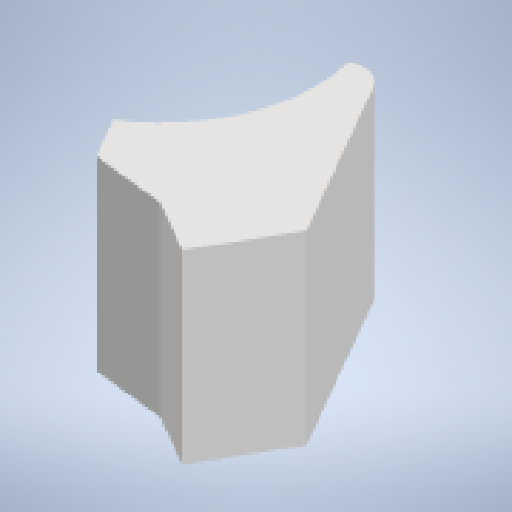
# Autodesk Inventor part: base_backwall_setter_under
Saved by Autodesk Inventor 2024.1 (Build 281209000, 209)
## iProperties
Created: 2025-01-18
Part Number: base_backwall_setter_under
Material: 一般
Document SubType Name: Modeling
Designer: hibik
Density: 1 g/cm^3
Appearance: 既定
Author: hibik
Autodesk Inventor part; units mm, degrees
ref_plane "YZ Plane" through (0, 0, 0) normal (1, 0, 0) x (0, 1, 0)
ref_plane "XZ Plane" through (0, 0, 0) normal (0, 1, 0) x (-1, 0, 0)
ref_plane "XY Plane" through (0, 0, 0) normal (0, 0, 1) x (1, 0, 0)
sketch "スケッチ2" plane through (0, 0, 0) normal (0, 1, 0) x (-1, 0, 0)
  line L0 (0, 0) -> (-8.6603, -15)
  line L1 (-8.6603, -15) -> (11.3397, -49.641)
  line L2 (73.7428, 0) -> (-22.3941, 0) projected
  line L3 (11.3397, -49.641) -> (5.9252, -52.7671) construction
  line L4 (0, 0) -> (-6.6711, 3.8516) construction
  line L5 (11.3397, -49.641) -> (24.3301, -42.141)
  line L6 (24.3301, -42.141) -> (0, 0)
  line L7 (0, 0) -> (8.2272, -4.75)
  line L8 (8.2272, -4.75) -> (-3.1754, -24.5)
  line L9 (-2.5935, -25.5079) -> (9.1002, -5.254)
  line L10 (9.1002, -5.254) -> (8.2272, -4.75)
  line L11 (-3.1754, -24.5) -> (2.5403, -27.8)
  line L12 (2.5403, -27.8) -> (12.2903, -10.9125)
  line L13 (12.2903, -10.9125) -> (6.5746, -7.6125)
  line L14 (6.5746, -7.6125) -> (-3.1754, -24.5)
  line L15 (11.3397, -49.641) -> (31.9282, -37.7543)
  line L16 (31.9282, -37.7543) -> (38.6416, -26.1264)
  line L17 (6.3397, -40.9808) -> (21.9282, -31.9808) construction
  line L18 (21.9282, -31.9808) -> (31.9282, -37.7543)
  line L19 (12.2903, -10.9125) -> (38.6416, -26.1264)
  line L20 (38.6416, -26.1264) -> (3.5066, -26.1264)
  line L21 (0, 0) -> (21.3397, 36.9615)
  line L22 (21.3397, 36.9615) -> (15.2136, 40.4985)
  line L23 (-0.5996, -1.0385) -> (60.009, -1.0385)
  circle A0 centre (21.3397, -13.5385) radius 12.5 construction
  circle A1 centre (21.3397, -13.5385) radius 10.5 construction
  circle A2 centre (20.5151, -34.5223) radius 10.5 construction
  circle A3 centre (20.5151, -34.5223) radius 11.5 construction
  circle A4 centre (20.5151, -34.5223) radius 12.5
  line L24 (8.3719, -37.4876) -> (11.3397, -49.641)
  line L25 (-2.3094, -23) -> (12.6388, -48.891)
  point P0 (9.2953, -16.1)
  point P1 (7.4475, -8.1165)
  point P2 (-2.3025, -25.004)
  point P3 (15.0841, -26.1264)
  point P4 (11.2545, -26.1264)
  point P5 (6.0668, -10.5079)
  point P6 (13.8325, -23.9586)
  point P7 (10.0702, -44.4421)
  point P8 (-1.7275, -24.0079)
  dimension "d34" = 25
  dimension "d11" = 60
  dimension "d12" = 60
  dimension "d13" = 40
  dimension "d15" = 15
  dimension "d16" = 9.5
  dimension "d17" = 1.0079
  dimension "d18" = 19.5
  dimension "d19" = 6.6
  dimension "d24" = 18
  dimension "d25" = 30
  dimension "d26" = 60
  dimension "d28" = 60
  dimension "d29" = 38
  dimension "d30" = 25
  dimension "d31" = 21
  dimension "d32" = 21
  dimension "d33" = 23
  dimension "d40" = 1.5
  constraints: 51 end point, 9 perpendicular, 7 point on line, 5 collinear, 5 parallel, 4 centre point, 3 coincident, 2 horizontal, 2 tangent, 1 equal radius, 1 vertical alignment, 4 other
  measures "d11" angle of L2 L0
  measures "d12" angle of L0 L1
  measures "d13" distance from line of L0.end L3
  measures "d15" distance between parallel lines of L1 L6
  measures "d16" distance between parallel lines of L0 L8
  measures "d17" distance between parallel lines of L8 L9
  measures "d18" distance between parallel lines of L11 L13
  measures "d19" distance between parallel lines of L14 L12
  measures "d24" distance from line of L17.end L1
  measures "d25" distance from line of L0.end L17
  measures "d26" angle of L17 L18
  measures "d28" distance from line of L0.end L22
  measures "d29" distance from line of L21.end L23
  measures "d30" diameter of A0
  measures "d31" diameter of A1
  measures "d32" diameter of A2
  measures "d33" diameter of A3
  measures "d40" distance between parallel lines of L1 L25
extrude "押し出し4" add sketch "スケッチ2" along normal blind 15 contours L6 L12 L11 L25 L9 | L6 A4 L20 L12 | L11 L12 L20 A4 L24 L25
fillet "フィレット1" radius 2 1 edges at (-10.0702, 7.5, -44.4421)
sketch "スケッチ3" plane through (0, 15, 0) normal (0, 1, 0) x (1, 0, 0)
  ellipse E0 centre (-16.5607, 22.817) end of major axis (-18.0607, 20.2189) minor radius 2.9999 (-18.4056, 20.4514) -> (-17.74, 20.0585) ccw projected
  ellipse E1 centre (-20.6882, 13.1623) end of major axis (-16.9382, 19.6575) minor radius 7.4997 (-13.3193, 14.5576) -> (-17.74, 20.0585) ccw projected
  line L0 (-13.3193, 14.5576) -> (-11.4591, 4.7323) projected
  line L1 (-11.4591, 4.7323) -> (-7.1359, 7.9366) projected
  line L2 (-7.1359, 7.9366) -> (-2.1359, 16.5968) projected
  line L3 (-2.1359, 16.5968) -> (-6.4659, 19.0967) projected
  line L4 (-6.4659, 19.0967) -> (-18.4056, 20.4514) projected
  line L5 (-6.0668, 10.5079) -> (1.7275, 24.0079) projected
  line L6 (-1.9475, 17.6428) -> (-6.1462, 20.0669)
  line L7 (-6.1462, 20.0669) -> (-11.9669, 20.7273)
  line L8 (-13.8325, 23.9586) -> (-6.0668, 10.5079) projected
  point P0 (0, 0)
  point P1 (2.5935, 25.5079)
  dimension "d36" = 1
  dimension "d37" = 1
  constraints: 4 end point, 2 parallel, 2 point on line, 1 perpendicular, 2 other
  measures "d36" distance between parallel lines of L3 L6
  measures "d37" distance between parallel lines of L4 L7
extrude "押し出し5" cut sketch "スケッチ3" against normal through all contours L8 L7 L6 L5 L3 L4 | L4 L3 L5 L8
equation "\"d37\" = d36"
